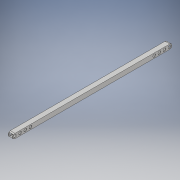
# Autodesk Inventor part: Support Pivs 25 uppermiddle
Saved by Autodesk Inventor 2018 (Build 220112000, 112)
## iProperties
Created: 2018-01-22
Part Number: Support Pivs 25 uppermiddle
Material: Generic
Document SubType Name: Modeling
Designer: lopez.xavier
Density: 1 g/cm^3
Appearance: Default
Author: lopez.xavier
Autodesk Inventor part; units mm, degrees
ref_plane "YZ Plane" through (0, 0, 0) normal (1, 0, 0) x (0, 1, 0)
ref_plane "XZ Plane" through (0, 0, 0) normal (0, 1, 0) x (-1, 0, 0)
ref_plane "XY Plane" through (0, 0, 0) normal (0, 0, 1) x (1, 0, 0)
sketch "Sketch1" plane through (0, 0, 0) normal (0, 0, 1) x (1, 0, 0)
  line L0 (0, 0) -> (25.4, 0)
  line L1 (25.4, 0) -> (25.4, 25.4)
  line L2 (25.4, 25.4) -> (0, 25.4)
  line L3 (0, 25.4) -> (0, 0)
  dimension "d0" = 25.4
  dimension "d1" = 25.4
  constraints: 8 end point, 2 parallel, 1 horizontal, 1 perpendicular
  measures "d0" distance of L1.end L2.end
  measures "d1" distance of L0.end L1.end
extrude "Extrusion1" add sketch "Sketch1" along normal blind 863.6
fillet "Fillet1" radius 12.7 4 edges at (12.7, 25.4, 863.6) (12.7, 0, 863.6) (12.7, 25.4, 0) (12.7, 0, 0)
sketch "Sketch2" plane through (0, 0, 0) normal (0, 0, 1) x (1, 0, 0)
  line L0 (22.86, 22.86) -> (2.54, 22.86)
  line L1 (2.54, 22.86) -> (2.54, 2.54)
  line L2 (2.54, 2.54) -> (22.86, 2.54)
  line L3 (22.86, 2.54) -> (22.86, 22.86)
  line L4 (0, 25.4) -> (25.4, 25.4) projected
  line L5 (0, 0) -> (0, 25.4) projected
  line L6 (25.4, 0) -> (0, 0) projected
  line L7 (25.4, 25.4) -> (25.4, 0) projected
  dimension "d5" = 2.54
  dimension "d6" = 2.54
  dimension "d7" = 2.54
  dimension "d8" = 2.54
  constraints: 8 end point, 2 parallel, 1 horizontal, 1 perpendicular
  measures "d5" distance between parallel lines of L4 L0
  measures "d6" distance between parallel lines of L5 L1
  measures "d7" distance between parallel lines of L6 L2
  measures "d8" distance between parallel lines of L7 L3
extrude "Extrusion2" cut sketch "Sketch2" along normal blind 1016 contours L3 L2 L1 L0
sketch "Sketch3" plane through (0, 12.7, 12.7) normal (-1, 0, 0) x (0, 0, 1)
  circle A0 centre (0, 0) radius 7.8422
  circle A1 centre (27.94, 0) radius 7.8422
  circle A2 centre (55.88, 0) radius 7.8422
  circle A3 centre (83.82, 0) radius 7.8423
  circle A4 centre (838.2, 0) radius 7.8423
  circle A5 centre (810.26, 0) radius 7.8422
  circle A6 centre (782.32, 0) radius 7.8422
  circle A7 centre (754.38, 0) radius 7.8423
  line L0 (0, 12.7) -> (838.2, 12.7)
  arc A8 (0, 12.7) -> (0, -12.7) centre (0, 0) ccw
  arc A9 (838.2, -12.7) -> (838.2, 12.7) centre (838.2, 0) ccw
  point P0 (-12.7, -12.7)
  dimension "d11" = 15.6845
  dimension "d12" = 15.6845
  dimension "d13" = 15.6845
  dimension "d14" = 15.6845
  dimension "d15" = 15.6845
  dimension "d16" = 15.6845
  dimension "d17" = 15.6845
  dimension "d18" = 15.6845
  dimension "d19" = 12.7
  dimension "d20" = 12.7
  dimension "d21" = 12.7
  dimension "d22" = 12.7
  dimension "d23" = 12.7
  dimension "d24" = 12.7
  dimension "d25" = 12.7
  dimension "d26" = 12.7
  dimension "d27" = 0
  dimension "d28" = 27.94
  dimension "d29" = 27.94
  dimension "d30" = 27.94
  dimension "d31" = 0
  dimension "d32" = 27.94
  dimension "d33" = 27.94
  dimension "d34" = 27.94
  constraints: 8 centre point
  measures "d11" diameter of A0
  measures "d12" diameter of A1
  measures "d13" diameter of A2
  measures "d14" diameter of A3
  measures "d15" diameter of A4
  measures "d16" diameter of A5
  measures "d17" diameter of A6
  measures "d18" diameter of A7
  measures "d19" distance from line of L0 A4.centre
  measures "d20" distance from line of L0 A5.centre
  measures "d21" distance from line of L0 A6.centre
  measures "d22" distance from line of L0 A7.centre
  measures "d23" distance from line of L0 A0.centre
  measures "d24" distance from line of L0 A1.centre
  measures "d25" distance from line of L0 A2.centre
  measures "d26" distance from line of L0 A3.centre
  measures "d27" distance of A8.centre A0.centre
  measures "d28" distance of A0.centre A1.centre
  measures "d29" distance of A1.centre A2.centre
  measures "d30" distance of A2.centre A3.centre
  measures "d31" distance of A9.centre A4.centre
  measures "d32" distance of A4.centre A5.centre
  measures "d33" distance of A5.centre A6.centre
  measures "d34" distance of A6.centre A7.centre
extrude "Extrusion3" cut sketch "Sketch3" against normal blind 25.4
equation "\"d29\" = d28"
equation "\"d30\" = d28"
equation "\"d33\" = d32"
equation "\"d34\" = d32"
body "Solid1"
